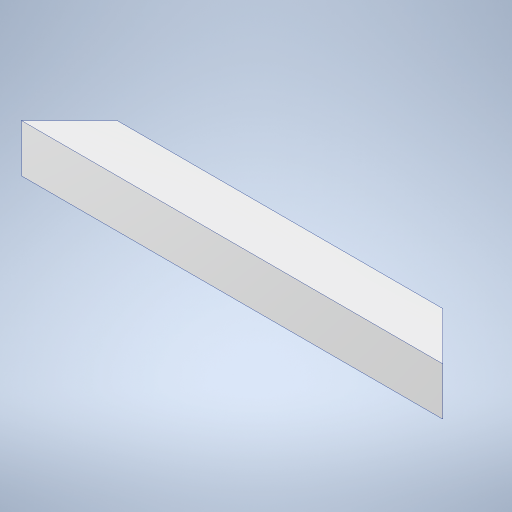
# Autodesk Inventor part: P406
Saved by Autodesk Inventor 2023 (Build 270158000, 158)
## iProperties
Created: 2022-08-30
Part Number: P406
Material: Aluminum 6061
Document SubType Name: Modeling
Designer: D.C. Eksteen
Density: 2.7 g/cm^3
Appearance: Aluminum - Flat
Author: D.C. Eksteen
Title: PLATFORM TUBE
Autodesk Inventor part; units mm, degrees
ref_plane "YZ Plane" through (0, 0, 0) normal (1, 0, 0) x (0, 1, 0)
ref_plane "XZ Plane" through (0, 0, 0) normal (0, 1, 0) x (-1, 0, 0)
ref_plane "XY Plane" through (0, 0, 0) normal (0, 0, 1) x (1, 0, 0)
sketch "Sketch1" plane through (0, 0, 0) normal (1, 0, 0) x (0, 1, 0)
  line L0 (0, 0) -> (25, 0)
  line L1 (25, 0) -> (25, -25)
  line L2 (25, -25) -> (0, -25)
  line L3 (0, -25) -> (0, 0)
  line L4 (22, -22) -> (22, -3)
  line L5 (22, -3) -> (3, -3)
  line L6 (3, -3) -> (3, -22)
  line L7 (3, -22) -> (22, -22)
  dimension "d0" = 25
  dimension "d1" = 25
  dimension "d2" = 3
  constraints: 16 end point, 4 parallel, 2 perpendicular, 1 horizontal, 3 other
  measures "d0" distance of L1.end L2.end
  measures "d1" distance of L0.end L1.end
  measures "d2" distance between parallel lines of L1 L4
extrude "Extrusion1" add sketch "Sketch1" along normal blind 220
sketch "Sketch2" plane through (0, 25, 0) normal (0, 1, 0) x (1, 0, 0)
  line L0 (0, 25) -> (0, 0) projected
  line L1 (0, 0) -> (220, 0) projected
  line L2 (220, 25) -> (220, 0) projected
  line L3 (0, 25) -> (220, 25) projected
  line L4 (0, 0) -> (220, 0) projected
  line L5 (0, 0) -> (25, 25)
  line L6 (0, 25) -> (220, 25) projected
  line L7 (220, 0) -> (220, 25) projected
  line L8 (220, 0) -> (195, 25)
  dimension "d5" = 45
  dimension "d6" = 45
  constraints: 4 end point, 2 point on line
  measures "d5" angle of L1 L5
  measures "d6" angle of L1 L8
extrude "Extrusion2" cut sketch "Sketch2" against normal blind 110 contours L3 L5 L0 | L8 L3 L2
body "Solid1"
